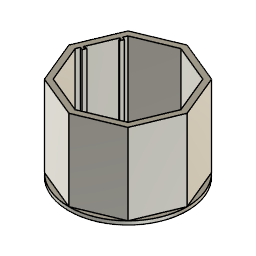
RootModule_sample (Autodesk Fusion 360 design; units mm, degrees)
part number: 2026-05-14-22-32-52-838
Autodesk Fusion 360 part; units mm, degrees
note: some values were not read from the file. Set by a fixed rule: which sketch regions a step uses.
sketch "Sketch1" plane through (0, 0, 0) normal (0, 0, 1) x (1, 0, 0)
  circle A0 centre (0, 0) radius 47.5
  dimension "d1" = 95
  constraint coincident A0.centre origin
  measures "d1" diameter of A0
extrude "Extrude1" add sketch "Sketch1" along normal blind 3
sketch "Sketch4" plane through (0, 0, 3) normal (0, 0, 1) x (-1, 0, 0)
  circle A0 centre (0, 0) radius 47.5
  line L0 (-47.5, 0) -> (-33.5876, -33.5876)
  line L1 (-33.5876, -33.5876) -> (0, -47.5)
  line L2 (0, -47.5) -> (33.5876, -33.5876)
  line L3 (33.5876, -33.5876) -> (47.5, 0)
  line L4 (47.5, 0) -> (33.5876, 33.5876)
  line L5 (33.5876, 33.5876) -> (0, 47.5)
  line L6 (0, 47.5) -> (-33.5876, 33.5876)
  line L7 (-33.5876, 33.5876) -> (-47.5, 0)
  dimension "d5" = 47.5
  constraint coincident A0.centre origin
  measures "d5" distance of L0.start A0.centre
extrude "Extrude2" add sketch "Sketch4" along normal blind 65 contours L0 L1 L2 L3 L4 L5 L6 L7
sketch "Sketch5" plane through (0, 0, 68) normal (0, 0, 1) x (-1, 0, 0)
  line L0 (-33.5876, 33.5876) -> (-47.5, 0)
  line L1 (-47.5, 0) -> (-33.5876, -33.5876)
  line L2 (-33.5876, -33.5876) -> (0, -47.5)
  line L3 (0, -47.5) -> (33.5876, -33.5876)
  line L4 (33.5876, -33.5876) -> (47.5, 0)
  line L5 (47.5, 0) -> (33.5876, 33.5876)
  line L6 (33.5876, 33.5876) -> (0, 47.5)
  line L7 (0, 47.5) -> (-33.5876, 33.5876)
  line L8 (42.5, 0) -> (30.052, 30.052)
  line L9 (30.052, 30.052) -> (0, 42.5)
  line L10 (0, 42.5) -> (-30.052, 30.052)
  line L11 (-30.052, 30.052) -> (-42.5, 0)
  line L12 (-42.5, 0) -> (-30.052, -30.052)
  line L13 (-30.052, -30.052) -> (0, -42.5)
  line L14 (0, -42.5) -> (30.052, -30.052)
  line L15 (30.052, -30.052) -> (42.5, 0)
  dimension "d8" = 42.5
  measures "d8" distance of L8.start origin
extrude "Extrude3" cut sketch "Sketch5" against normal blind 65 contours L8 L9 L10 L11 L12 L13 L14 L15
sketch "Sketch6" plane through (-36.276, 15.026, 0) normal (0.92388, -0.382683, 0) x (0.382683, 0.92388, 0)
  line L0 (16.264, 68) -> (-16.264, 68)
  line L1 (-16.264, 68) -> (-16.264, 3)
  line L2 (-16.264, 3) -> (16.264, 3)
  line L3 (16.264, 3) -> (16.264, 68)
  line L4 (-16.264, 68) -> (16.264, 68)
  line L5 (0, 68) -> (-11, 68)
  line L6 (0, 68) -> (11, 68)
  line L7 (11, 68) -> (13, 68)
  line L8 (13, 68) -> (13, 3)
  line L9 (13, 3) -> (11, 3)
  line L10 (-11, 68) -> (-13, 68)
  line L11 (-13, 68) -> (-13, 3)
  line L12 (-13, 3) -> (-11, 3)
  line L13 (-13, 68) -> (-11.25, 68)
  line L14 (-11.25, 68) -> (-11.25, 3)
  line L15 (-11.25, 3) -> (-13, 3)
  line L16 (-13, 3) -> (-13, 68)
  line L17 (13, 68) -> (11.25, 68)
  line L18 (11.25, 68) -> (11.25, 3)
  line L19 (11.25, 3) -> (13, 3)
  line L20 (13, 3) -> (13, 68)
  dimension "d11" = 11
  dimension "d12" = 11
  dimension "d13" = 2
  dimension "d14" = 65
  dimension "d25" = 1.75
  dimension "d26" = 65
  dimension "d27" = 1.75
  dimension "d28" = 65
  constraint coincident L0.end L1.start
  constraint coincident L0.start L3.end
  constraint midpoint L4 L5.start
  constraint parallel L0 L5
  constraint parallel L4 L6
  constraint horizontal L7
  constraint vertical L8
  constraint horizontal L9
  constraint coincident L2 L8.end
  constraint horizontal L10
  constraint vertical L11
  constraint horizontal L12
  constraint horizontal L13
  constraint vertical L14
  constraint horizontal L15
  constraint vertical L16
  constraint horizontal L17
  constraint vertical L18
  constraint horizontal L19
  constraint vertical L20
  measures "d11" distance of L5.start L5.end
  measures "d12" distance of L5.start L6.end
  measures "d13" distance of L6.end L7.end
  measures "d14" distance of L5.end L12.end
  measures "d25" distance of L10.end L13.end
  measures "d26" distance of L10.end L11.end
  measures "d27" distance of L7.end L17.end
  measures "d28" distance of L7.end L8.end
extrude "Extrude4" add sketch "Sketch6" along normal blind 1.5 contours L0 L2 L4 L7 L8 L9 L17 L18 L19 L20 | L0 L2 L4 L10 L11 L12 L13 L14 L15 L16
sketch "Sketch7" plane through (-34.8902, 14.452, 0) normal (0.92388, -0.382683, 0) x (0.382683, 0.92388, 0)
  line L0 (-11.25, 68) -> (-13, 68)
  line L1 (-13, 68) -> (-13, 3)
  line L2 (-13, 3) -> (-11.25, 3)
  line L3 (-13, 68) -> (-10, 68)
  line L4 (-10, 68) -> (-10, 3)
  line L5 (-10, 3) -> (-13, 3)
  line L6 (-13, 3) -> (-13, 68)
  line L7 (-11.25, 3) -> (-11.25, 68)
  dimension "d17" = 3
  dimension "d18" = 65
  constraint horizontal L3
  constraint vertical L4
  constraint horizontal L5
  constraint vertical L6
  constraint coincident L0.end L1.start
  measures "d17" distance of L0.end L3.end
  measures "d18" distance of L0.end L1.end
extrude "Extrude5" add sketch "Sketch7" along normal blind 1
sketch "Sketch8" plane through (-34.8902, 14.452, 0) normal (0.92388, -0.382683, 0) x (0.382683, 0.92388, 0)
  line L0 (11.25, 3) -> (13, 3)
  line L1 (13, 68) -> (11.25, 68)
  line L2 (13, 68) -> (10, 68)
  line L3 (10, 68) -> (10, 3)
  line L4 (10, 3) -> (13, 3)
  line L5 (13, 3) -> (13, 68)
  line L6 (13, 3) -> (13, 68)
  line L7 (11.25, 68) -> (11.25, 3)
  dimension "d21" = 3
  dimension "d22" = 65
  constraint horizontal L2
  constraint vertical L3
  constraint horizontal L4
  constraint vertical L5
  constraint coincident L1.start L2.start
  measures "d21" distance of L1.start L2.end
  measures "d22" distance of L1.start L0.end
extrude "Extrude6" add sketch "Sketch8" along normal blind 1
